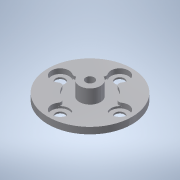
# Autodesk Inventor part: 足首_独立ピッチ_1_2
Saved by Autodesk Inventor 2020 (Build 240168000, 168)
## iProperties
Created: 2016-05-04
Part Number: 足首_独立ピッチ_1_2
Material: アルミニウム 2014-T4
Document SubType Name: Modeling
Designer: hiroaki
Density: 2.8 g/cm^3
Appearance: サテン
Mass: 1.76953 g
Surface Area: 11.344 cm^2
Volume: 0.631975 cm^3
Category: 足首
Author: hiroaki
Autodesk Inventor part; units mm, degrees
ref_plane "YZ Plane" through (0, 0, 0) normal (1, 0, 0) x (0, 1, 0)
ref_plane "XZ Plane" through (0, 0, 0) normal (0, 1, 0) x (-1, 0, 0)
ref_plane "XY Plane" through (0, 0, 0) normal (0, 0, 1) x (1, 0, 0)
sketch "スケッチ1" plane through (0, 0, 0) normal (0, 0, 1) x (1, 0, 0)
  circle A0 centre (0, 8.5) radius 1.35
  circle A1 centre (0, 0) radius 1.25
  circle A2 centre (0, 0) radius 3
  circle A3 centre (0, 0) radius 6.05
  circle A4 centre (0, 8.5) radius 2.5
  circle A5 centre (-8.5, 0) radius 1.35
  circle A6 centre (-8.5, 0) radius 2.5
  circle A7 centre (0, -8.5) radius 1.35
  circle A8 centre (0, -8.5) radius 2.5
  circle A9 centre (8.5, 0) radius 1.35
  circle A10 centre (8.5, 0) radius 2.5
  circle A11 centre (0, 0) radius 6 construction
  circle A12 centre (0, 0) radius 12
  point P0 (6.0354, -0.4195)
  point P1 (6.0354, 0.4195)
  point P2 (0.4195, 6.0354)
  point P3 (-0.4195, 6.0354)
  point P4 (-6.0354, 0.4195)
  point P5 (-6.0354, -0.4195)
  point P6 (-0.4195, -6.0354)
  point P7 (0.4195, -6.0354)
  dimension "d0" = 2.7
  dimension "d1" = 8.5
  dimension "d3" = 2.5
  dimension "d33" = 6
  dimension "d55" = 12.1
  dimension "d58" = 5
  dimension "d61" = 360
  dimension "d66" = 12
  dimension "d71" = 24
  constraints: 13 centre point, 9 coincident, 1 vertical alignment, 17 other
  measures "d0" diameter of A0
  measures "d1" distance of point (0, 0) A0.centre
  measures "d3" diameter of A1
  measures "d33" diameter of A2
  measures "d55" diameter of A3
  measures "d58" diameter of A4
  measures "d66" diameter of A11
  measures "d71" diameter of A12
extrude "押し出し1" add sketch "スケッチ1" along normal blind 5 contours A2
extrude "押し出し2" add sketch "スケッチ1" along normal blind 0.45 contours A1 | A2 | A3 A10 | A3 A10 | A4 A3 | A3 A4 | A8 A3 | A3 A8 | A6 A3 | A3 A6
extrude "押し出し3" add sketch "スケッチ1" along normal blind 1.85 contours A12
extrude "押し出し4" add sketch "スケッチ1" along normal blind 1 contours A10 A3 A8 A6 A4
fillet "フィレット2" radius 1 8 edges at (-6.0354, -0.4195, 1.425) (-6.0354, 0.4195, 1.425) (-0.4195, -6.0354, 1.425) (0.4195, -6.0354, 1.425) (6.0354, -0.4195, 1.425) (6.0354, 0.4195, 1.425) (0.4195, 6.0354, 1.425) (-0.4195, 6.0354, 1.425)
